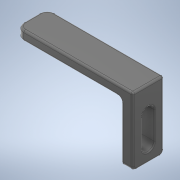
# Autodesk Inventor part: Leg Shelf
Saved by Autodesk Inventor 2020 (Build 240168000, 168)
## iProperties
Created: 2020-02-14
Part Number: Leg Shelf
Material: ABS Plastic
Document SubType Name: Modeling
Designer: Ishaan
Density: 1.06 g/cm^3
Appearance: Smooth - Black
Author: Ishaan
Autodesk Inventor part; units mm, degrees
ref_plane "YZ Plane" through (0, 0, 0) normal (1, 0, 0) x (0, 1, 0)
ref_plane "XZ Plane" through (0, 0, 0) normal (0, 1, 0) x (-1, 0, 0)
ref_plane "XY Plane" through (0, 0, 0) normal (0, 0, 1) x (1, 0, 0)
sketch "Sketch1" plane through (0, 0, 0) normal (0, 1, 0) x (-1, 0, 0)
  line L0 (-1.5, -4) -> (1.5, -4)
  line L1 (1.5, -4) -> (1.5, 4)
  line L2 (1.5, 4) -> (-1.5, 4)
  line L3 (-1.5, 4) -> (-1.5, -4)
  line L4 (-1.5, -4) -> (1.5, 4) construction
  line L5 (1.5, -4) -> (-1.5, 4) construction
  line L6 (1.5, 3) -> (4.5, 0)
  line L7 (4.5, 0) -> (1.5, -3)
  point P0 (0, 0)
  point P1 (0, 0)
  dimension "d0" = 3
  dimension "d1" = 8
  dimension "d2" = 1
  dimension "d3" = 3
  constraints: 16 end point, 3 midpoint, 2 parallel, 2 perpendicular, 2 point on line, 1 horizontal, 1 horizontal alignment
  measures "d0" distance of L2.end L1.end
  measures "d1" distance of L1.end L0.end
  measures "d2" distance from line of L6.start L2
  measures "d3" distance from line of L1 L6.end
extrude "Extrusion1" add sketch "Sketch1" along normal blind 15
sketch "Sketch2" plane through (1.5, 0, 4) normal (1, 0, 0) x (0, 0, -1)
  line L0 (0, 15) -> (8, 15) projected
  line L1 (4, 11) -> (4, 4) construction
  line L2 (7, 0) -> (7, 15) projected
  line L3 (2.4, 11) -> (2.4, 4)
  line L4 (5.6, 4) -> (5.6, 11)
  arc A0 (5.6, 11) -> (2.4, 11) centre (4, 11) ccw
  arc A1 (2.4, 4) -> (5.6, 4) centre (4, 4) ccw
  line L5 (0, 0) -> (8, 0) projected
  point P0 (4, 0)
  point P1 (4, 15)
  point P2 (4, 7.5)
  dimension "d6" = 4
  dimension "d7" = 3.2
  dimension "d8" = 4
  dimension "d53" = 7
  constraints: 8 end point, 4 point on circle, 4 tangent, 2 centre point, 2 midpoint, 2 parallel, 1 vertical alignment
  measures "d6" distance from line of L1.start L0
  measures "d7" diameter of A1
  measures "d8" distance from line of L1.end L5
  measures "d53" distance of L1.start L1.end
extrude "Extrusion2" cut sketch "Sketch2" against normal through all
sketch "Sketch3" plane through (0, 15, 0) normal (0, 1, 0) x (1, 0, 0)
  line L0 (-4.5, 0) -> (-1.5, -3) projected
  line L1 (-1.5, -3) -> (-1.5, -4) projected
  line L2 (-1.5, -4) -> (1.5, -4) projected
  line L3 (1.5, -4) -> (1.5, 4) projected
  line L4 (1.5, 4) -> (-1.5, 4) projected
  line L5 (-1.5, 4) -> (-1.5, 3) projected
  line L6 (-1.5, 3) -> (-4.5, 0) projected
  line L7 (1.5, 4) -> (-28.5, 4)
  line L8 (-28.5, 4) -> (-28.5, -4)
  line L9 (-28.5, -4) -> (1.5, -4)
  line L10 (1.5, -4) -> (1.5, 4)
  line L11 (-16.5, 4) -> (-10.5, 4)
  line L12 (-10.5, 4) -> (-10.5, 8)
  line L13 (-10.5, 8) -> (-16.5, 8)
  line L14 (-16.5, 8) -> (-16.5, 4)
  line L15 (-16.5, 8) -> (-17.5718, 4)
  line L16 (-10.5, 8) -> (-9.4282, 4)
  point P0 (0, 0)
  point P1 (-13.5, 4)
  dimension "d11" = 30
  dimension "d30" = 6
  dimension "d31" = 12
  dimension "d32" = 30
  dimension "d52" = 4
  constraints: 20 end point, 4 parallel, 3 point on line, 2 horizontal, 2 midpoint, 2 perpendicular, 1 collinear, 1 equal length
  measures "d11" distance of L9.end L8.end
  measures "d30" distance of L13.end L12.end
  measures "d31" distance between parallel lines of L13 L9
  measures "d32" angle of L16 L15
  measures "d52" distance of L13.end L11.start
extrude "Extrusion3" add sketch "Sketch3" along normal blind 2.5 contours L6 L5 L4 L3 L2 L1 L0 | L0 L1 L9 L8 L7 L5 L6
sketch "Sketch5" plane through (0, 17.5, 0) normal (0, 1, 0) x (1, 0, 0)
  line L0 (-16.5, 8) -> (-17.5718, 4) projected
  line L1 (-10.5, 8) -> (-16.5, 8) projected
  line L2 (-9.4282, 4) -> (-10.5, 8) projected
  line L3 (-16.6705, 3.5) -> (-15.7327, 7)
  line L4 (-15.7327, 7) -> (-11.2673, 7)
  line L5 (-11.2673, 7) -> (-10.3295, 3.5)
  line L6 (-16.6705, 3.5) -> (-17.7058, 3.5)
  line L7 (-16.5, 8) -> (-17.5718, 4) projected
  line L8 (-9.4282, 4) -> (-10.5, 8) projected
  line L9 (-10.3295, 3.5) -> (-9.2942, 3.5)
  line L10 (-1.5, 4) -> (-28.5, 4) projected
  line L11 (-17.7058, 3.5) -> (-17.5718, 4)
  line L12 (-9.4282, 4) -> (-9.2942, 3.5)
  line L13 (1.5, 4) -> (-28.5, 4) projected
  point P0 (0, 0)
  dimension "d33" = 1
  dimension "d44" = 0.5
  constraints: 14 end point, 3 collinear, 1 parallel, 2 other
  measures "d33" distance between parallel lines of L1 L4
  measures "d44" distance between parallel lines of L10 L6
extrude "Extrusion5" [suppressed]
sketch "Sketch6" plane through (-10.5, 15, -8) normal (0, 0, -1) x (-1, 0, 0)
  line L0 (0, 0) -> (6, 0) projected
  line L1 (6, 0) -> (6, 2.5) projected
  line L2 (0, 0) -> (0, 2.5) projected
  line L3 (0, 2.5) -> (6, 2.5) projected
  point P0 (-10.5, -15)
  point P1 (3, 3.5)
  point P2 (3, 3)
  constraints: 1 vertical alignment
hole "Hole1" [suppressed]
fillet "Fillet10" [suppressed]
fillet "Fillet11" [suppressed]
fillet "Fillet12" [suppressed]
fillet "Fillet15" [suppressed]
fillet "Fillet13" [suppressed]
fillet "Fillet5" radius 1 4 edges at (-4.5, 1.2, 0) (-4.5, 13.8, 0) (-1.5, 7.5, -3) (-1.5, 7.5, 3)
fillet "Fillet16" radius 2 2 edges at (-28.5, 16.25, 4) (-28.5, 16.25, -4)
fillet "Fillet7" radius 1 2 edges at (0, 0, -4) (0, 0, 4)
fillet "Fillet6" radius 1 7 edges at (-1.5761, 15, -3.0315) (-2.7929, 15, -1.7071) (-4.0858, 15, 0) (-2.7929, 15, 1.7071) (-1.5761, 15, 3.0315) (-1.5, 15, 3.7071) (-1.5, 15, -3.7071)
fillet "Fillet14" [suppressed]
fillet "Fillet8" radius 0.5 22 edges at (-1.7929, 14.7071, -4) (-14.5, 15, -4) (-1.5, 0.4588, -3.8409) (-1.6782, 0, -2.8444) (-2.7929, 0, -1.7071) (-4.0858, 0, 0) (-2.7929, 0, 1.7071) (-1.6782, 0, 2.8444) (-1.5, 0.4588, 3.8409) (-1.5, 7.5, 4) (-1.5, 7.5, -4) (1.5, 9.25, 4) (1.5, 0.2929, 3.7071) (1.5, 0, 0) (1.5, 0.2929, -3.7071) (1.5, 9.25, -4) (-14.5, 15, 4) (-28.5, 15, 0) (-12.5, 17.5, 4) (1.5, 17.5, 0) (-28.5, 17.5, 0) (-12.5, 17.5, -4)
fillet "Fillet9" radius 0.25 12 edges at (-4.0858, 12.6, 0) (-3.1414, 11.8452, 1.3586) (-2.9, 7.5, 1.6) (-3.1414, 3.1548, 1.3586) (-4.0858, 2.4, 0) (-3.1414, 3.1548, -1.3586) (-2.9, 7.5, -1.6) (-3.1414, 11.8452, -1.3586) (1.5, 2.4, 0) (1.5, 7.5, 1.6) (1.5, 12.6, 0) (1.5, 7.5, -1.6)
equation "\"d8\" = d6"
body "Solid1"
